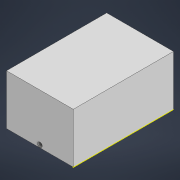
# Autodesk Inventor part: Box 1
Saved by Autodesk Inventor 2022 (Build 260153000, 153)
## iProperties
Created: 2021-07-26
Part Number: Box 1
Material: Generic
Document SubType Name: Modeling
Designer: Siddhant
Density: 1 g/cm^3
Appearance: Default
Author: Siddhant
Autodesk Inventor part; units mm, degrees
ref_plane "YZ Plane" through (0, 0, 0) normal (1, 0, 0) x (0, 1, 0)
ref_plane "XZ Plane" through (0, 0, 0) normal (0, 1, 0) x (-1, 0, 0)
ref_plane "XY Plane" through (0, 0, 0) normal (0, 0, 1) x (1, 0, 0)
sketch "Sketch1" plane through (0, 0, 0) normal (0, 1, 0) x (-1, 0, 0)
  line L0 (0, 0) -> (100, 0)
  line L1 (100, 0) -> (100, -150)
  line L2 (100, -150) -> (0, -150)
  line L3 (0, -150) -> (0, 0)
  dimension "d0" = 100
  dimension "d1" = 150
  constraints: 8 end point, 2 parallel, 1 horizontal, 1 perpendicular
  measures "d0" distance of L1.end L2.end
  measures "d1" distance of L2.end L0.start
extrude "Extrusion1" add sketch "Sketch1" along normal blind 75
sketch "Sketch2" plane through (0, 0, -150) normal (0, 0, -1) x (-1, 0, 0)
  line L0 (0, 0) -> (100, 0) projected
  circle A0 centre (50, 4) radius 3.5
  constraints: 1 centre point
hole "Hole1" at (-50, 4, -150) direction (0, 0, 1) diameter 7 depth 8
sketch "Sketch3" plane through (-100, 0, 0) normal (0, 0, 1) x (1, 0, 0)
  circle A0 centre (50, 4) radius 3.5 projected
  circle A1 centre (50, 4) radius 3.5
  point P0 (100, 0)
  constraints: 1 centre point, 1 coincident
hole "Hole2" at (-50, 4, 0) direction (0, 0, -1) diameter 7 depth 8
sketch "Sketch4" plane through (0, 0, 0) normal (0, -1, 0) x (1, 0, 0)
  point P0 (0, 0)
sketch "Sketch5" plane through (0, 0, 0) normal (0, -1, 0) x (1, 0, 0)
  line L0 (0, 0) -> (0, -150) projected
  line L1 (0, -75) -> (-100, -75)
  line L2 (-100, -150) -> (-100, 0) projected
  constraints: 2 end point, 2 midpoint
sketch "Sketch6" plane through (0, 0, 0) normal (0, -1, 0) x (1, 0, 0)
  circle A0 centre (-17.5284, -75) radius 15
  point P0 (0, 0)
  dimension "d20" = 30
  constraints: 1 centre point
  measures "d20" diameter of A0
hole "Hole3" at (-17.5284, 0, -75) direction (0, 1, 0) diameter 29 depth 15
body "Solid1"
